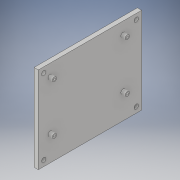
# Autodesk Inventor part: JetsonPlate
Saved by Autodesk Inventor 2019 (Build 230136000, 136)
## iProperties
Created: 2019-12-14
Part Number: JetsonPlate
Material: Generic
Document SubType Name: Modeling
Designer: james
Density: 1 g/cm^3
Appearance: Default
Author: james
Autodesk Inventor part; units mm, degrees
ref_plane "YZ Plane" through (0, 0, 0) normal (1, 0, 0) x (0, 1, 0)
ref_plane "XZ Plane" through (0, 0, 0) normal (0, 1, 0) x (-1, 0, 0)
ref_plane "XY Plane" through (0, 0, 0) normal (0, 0, 1) x (1, 0, 0)
sketch "Sketch1" plane through (0, 0, 0) normal (1, 0, 0) x (0, 1, 0)
  line L0 (60.8092, 49.7341) -> (-41.1908, 49.7341)
  line L1 (-41.1908, 49.7341) -> (-41.1908, -72.2659)
  line L2 (-41.1908, -72.2659) -> (60.8092, -72.2659)
  line L3 (60.8092, -72.2659) -> (60.8092, 49.7341)
  point P0 (0, 0)
  dimension "d0" = 122
  dimension "d1" = 102
  constraints: 8 end point, 2 parallel, 1 horizontal, 1 perpendicular
  measures "d0" distance of L2.end L0.start
  measures "d1" distance between parallel lines of L1 L3
extrude "Extrusion1" add sketch "Sketch1" along normal blind 5.08
sketch "Sketch2" plane through (5.08, 0, 0) normal (1, 0, 0) x (0, 0, -1)
  line L0 (-49.7341, 60.8092) -> (-49.7341, -41.1908) projected
  line L1 (72.2659, 60.8092) -> (-49.7341, 60.8092) projected
  point P0 (0, 0)
  point P1 (-35.7341, 46.8092)
  point P2 (50.2659, 46.8092)
  point P3 (50.2659, -11.1908)
  point P4 (-35.7341, -11.1908)
  dimension "d5" = 0
  dimension "d15" = 14
  dimension "d16" = 14
  dimension "d17" = 0
  dimension "d18" = 72
  dimension "d19" = 100
  dimension "d20" = 0
  dimension "d21" = 0
  measures "d5" horizontal distance of point (50.266, -11.191) point (50.266, 46.809)
  measures "d15" distance from line of L0 point (-35.734, 46.809)
  measures "d16" distance from line of L1 point (-35.734, 46.809)
  measures "d17" horizontal distance of point (-35.734, 46.809) point (-35.734, -11.191)
  measures "d18" distance from line of L1 point (-35.734, -11.191)
  measures "d19" distance from line of L0 point (50.266, 46.809)
  measures "d20" vertical distance of point (50.266, -11.191) point (-35.734, -11.191)
  measures "d21" vertical distance of point (-35.734, 46.809) point (50.266, 46.809)
hole "Hole1" at (5.08, 46.8092, 35.7341) at (5.08, 46.8092, -50.2659) at (5.08, -11.1908, -50.2659) at (5.08, -11.1908, 35.7341) direction (-1, 0, 0) diameter 2.0574 end through all clearance for "Flat Head Machine Screw (82)" size "#1" standard "Ansi Unified Screw Threads"
sketch "Sketch3" plane through (5.08, 0, 0) normal (1, 0, 0) x (0, 0, -1)
  circle A0 centre (-35.7341, 46.8092) radius 1.0287 projected
  circle A1 centre (-35.7341, 46.8092) radius 2.54
  circle A2 centre (50.2659, 46.8092) radius 1.0287 projected
  circle A3 centre (50.2659, 46.8092) radius 2.54
  circle A4 centre (50.2659, -11.1908) radius 1.0287 projected
  circle A5 centre (50.2659, -11.1908) radius 2.54
  circle A6 centre (-35.7341, -11.1908) radius 1.0287 projected
  circle A7 centre (-35.7341, -11.1908) radius 2.54
  point P0 (0, 0)
  dimension "d22" = 5.08
  dimension "d23" = 5.08
  dimension "d24" = 5.08
  dimension "d25" = 5.08
  constraints: 4 centre point, 4 coincident
  measures "d22" diameter of A1
  measures "d23" diameter of A3
  measures "d24" diameter of A5
  measures "d25" diameter of A7
extrude "Extrusion2" add sketch "Sketch3" along normal blind 5.08
sketch "Sketch4" plane through (5.08, 0, 0) normal (1, 0, 0) x (0, 0, -1)
  line L0 (-49.7341, 60.8092) -> (-49.7341, -41.1908) projected
  line L1 (72.2659, 60.8092) -> (-49.7341, 60.8092) projected
  point P0 (0, 0)
  point P1 (-43.3841, 54.4592)
  point P2 (65.8359, 54.4592)
  point P3 (-43.3841, -34.4408)
  point P4 (65.8359, -34.4408)
  dimension "d28" = 6.35
  dimension "d29" = 6.35
  dimension "d30" = 109.22
  dimension "d31" = 0
  dimension "d32" = 88.9
  dimension "d33" = 0
  dimension "d34" = 0
  dimension "d35" = 0
  measures "d28" distance from line of L0 point (-43.384, 54.459)
  measures "d29" distance from line of L1 point (-43.384, 54.459)
  measures "d30" distance of point (-43.384, 54.459) point (65.836, 54.459)
  measures "d31" vertical distance of point (-43.384, 54.459) point (65.836, 54.459)
  measures "d32" distance of point (-43.384, -34.441) point (-43.384, 54.459)
  measures "d33" horizontal distance of point (-43.384, 54.459) point (-43.384, -34.441)
  measures "d34" horizontal distance of point (65.836, -34.441) point (65.836, 54.459)
  measures "d35" vertical distance of point (-43.384, -34.441) point (65.836, -34.441)
hole "Hole2" at (5.08, 54.4592, 43.3841) at (5.08, 54.4592, -65.8359) at (5.08, -34.4408, 43.3841) at (5.08, -34.4408, -65.8359) direction (-1, 0, 0) diameter 5.1054 end through all clearance for "Flat Head Machine Screw (82)" size "#10" standard "Ansi Unified Screw Threads"
body "Solid1"
